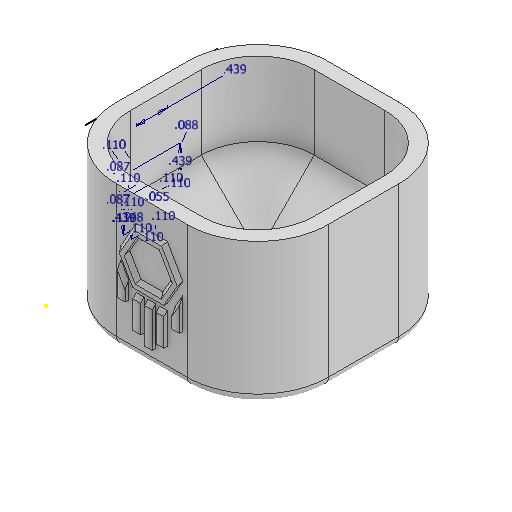
# Autodesk Inventor part: Hand Base
Saved by Autodesk Inventor 2025.1 (Build 291241020, 241B)
## iProperties
Created: 2025-01-03
Part Number: Hand Base
Material: Generic
Document SubType Name: Modeling
Designer: alexa
Density: 1 g/cm^3
Appearance: Default
Author: alexa
Autodesk Inventor part; units mm, degrees
ref_plane "YZ Plane" through (0, 0, 0) normal (1, 0, 0) x (0, 1, 0)
ref_plane "XZ Plane" through (0, 0, 0) normal (0, 1, 0) x (-1, 0, 0)
ref_plane "XY Plane" through (0, 0, 0) normal (0, 0, 1) x (1, 0, 0)
sketch "Sketch1" plane through (0, 0, 0) normal (0, 1, 0) x (-1, 0, 0)
  line L0 (0, 0) -> (-76.2, 0)
  line L1 (-76.2, 0) -> (-76.2, -76.2)
  line L2 (-76.2, -76.2) -> (0, -76.2)
  line L3 (0, -76.2) -> (0, 0)
  dimension "d0" = 76.2
  dimension "d1" = 76.2
  constraints: 8 end point, 2 parallel, 1 horizontal, 1 perpendicular
  measures "d0" distance of L2.end L0.start
  measures "d1" distance of L1.end L2.end
extrude "Extrusion1" add sketch "Sketch1" along normal blind 50.8
sketch "Sketch3" plane through (0, 0, 0) normal (0, -1, 0) x (1, 0, 0)
  line L0 (44.196, -54.102) -> (32.004, -54.102)
  line L1 (32.004, -54.102) -> (32.004, -22.098)
  line L2 (32.004, -22.098) -> (44.196, -22.098)
  line L3 (44.196, -22.098) -> (44.196, -54.102)
  line L4 (76.2, 0) -> (76.2, -76.2) projected
  line L5 (0, 0) -> (76.2, 0) projected
  line L6 (32.004, -40.132) -> (6.604, -40.132)
  line L7 (6.604, -40.132) -> (6.604, -36.068)
  line L8 (6.604, -36.068) -> (32.004, -36.068)
  line L9 (32.004, -36.068) -> (32.004, -40.132)
  point P0 (44.196, -38.1)
  point P1 (76.2, -38.1)
  point P2 (38.1, -22.098)
  point P3 (38.1, 0)
  point P4 (6.604, -38.1)
  point P5 (32.004, -38.1)
  dimension "d10" = 32.004
  dimension "d11" = 12.192
  dimension "d12" = 25.4
  dimension "d13" = 4.064
  constraints: 16 end point, 6 midpoint, 4 parallel, 2 horizontal, 2 horizontal alignment, 2 perpendicular, 1 point on line, 1 vertical alignment
  measures "d10" distance of L2.end L0.start
  measures "d11" distance of L0.start L0.end
  measures "d12" distance of L6.start L6.end
  measures "d13" distance of L6.end L7.end
extrude "Extrusion3" add sketch "Sketch3" along normal blind 6.35
sketch "Sketch4" plane through (0, -6.35, 0) normal (0, -1, 0) x (1, 0, 0)
  line L0 (43.942, -49.022) -> (32.258, -49.022)
  line L1 (32.258, -49.022) -> (32.258, -27.178)
  line L2 (32.258, -27.178) -> (43.942, -27.178)
  line L3 (43.942, -27.178) -> (43.942, -49.022)
  line L4 (44.196, -54.102) -> (44.196, -22.098) projected
  line L5 (32.004, -54.102) -> (44.196, -54.102) projected
  point P0 (0, 0)
  point P1 (32.258, -38.1)
  point P2 (44.196, -38.1)
  point P3 (38.1, -49.022)
  point P4 (38.1, -54.102)
  dimension "d16" = 21.844
  dimension "d17" = 11.684
  constraints: 8 end point, 4 midpoint, 2 parallel, 1 horizontal, 1 horizontal alignment, 1 perpendicular, 1 vertical alignment
  measures "d16" distance of L0.end L1.end
  measures "d17" distance between parallel lines of L1 L3
extrude "Extrusion4" add sketch "Sketch4" along normal blind 12.7
fillet "Fillet1" radius 25.4 4 edges at (0, 25.4, -76.2) (0, 25.4, 0) (76.2, 25.4, -76.2) (76.2, 25.4, 0)
sketch "Sketch5" plane through (0, 50.8, 0) normal (0, 1, 0) x (1, 0, 0)
  arc A0 (50.8, 0) -> (76.2, 25.4) centre (50.8, 25.4) ccw projected
  line L0 (76.2, 25.4) -> (76.2, 50.8) projected
  arc A1 (76.2, 50.8) -> (50.8, 76.2) centre (50.8, 50.8) ccw projected
  line L1 (50.8, 76.2) -> (25.4, 76.2) projected
  arc A2 (25.4, 76.2) -> (0, 50.8) centre (25.4, 50.8) ccw projected
  line L2 (0, 50.8) -> (0, 25.4) projected
  arc A3 (0, 25.4) -> (25.4, 0) centre (25.4, 25.4) ccw projected
  line L3 (25.4, 0) -> (50.8, 0) projected
  arc A4 (25.4, 71.12) -> (5.08, 50.8) centre (25.4, 50.8) ccw
  line L4 (25.4, 71.12) -> (50.8, 71.12)
  arc A5 (71.12, 50.8) -> (50.8, 71.12) centre (50.8, 50.8) ccw
  line L5 (71.12, 50.8) -> (71.12, 25.4)
  arc A6 (50.8, 5.08) -> (71.12, 25.4) centre (50.8, 25.4) ccw
  line L6 (50.8, 5.08) -> (25.4, 5.08)
  arc A7 (5.08, 25.4) -> (25.4, 5.08) centre (25.4, 25.4) ccw
  line L7 (5.08, 25.4) -> (5.08, 50.8)
  point P0 (0, 0)
  point P1 (38.1, 76.2)
  dimension "d21" = 5.08
  constraints: 8 end point, 8 point on circle, 4 centre point, 1 midpoint, 7 other
  measures "d21" distance from line of point (38.1, 76.2) L4
extrude "Extrusion5" cut sketch "Sketch5" against normal blind 45.72 contours L4 A5 L5 A6 L6 A7 L7 A4
fillet "Fillet2" radius 3.175 8 edges at (0, 0, -38.1) (7.4395, 0, -7.4395) (38.1, 0, 0) (68.7605, 0, -7.4395) (76.2, 0, -38.1) (68.7605, 0, -68.7605) (38.1, 0, -76.2) (7.4395, 0, -68.7605)
chamfer "Chamfer1" distance 19.05 angle 45 8 edges at (38.1, 5.08, -5.08) (11.0316, 5.08, -11.0316) (5.08, 5.08, -38.1) (11.0316, 5.08, -65.1684) (38.1, 5.08, -71.12) (65.1684, 5.08, -65.1684) (71.12, 5.08, -38.1) (65.1684, 5.08, -11.0316)
sketch "Sketch6" plane through (0, 50.8, -50.8) normal (-1, 0, 0) x (0, 0, 1)
  line L0 (7.2288, -10.0054) -> (18.3794, -10.0054)
  line L1 (18.3794, -10.0054) -> (23.9547, -19.6621)
  line L2 (23.9547, -19.6621) -> (18.3794, -29.3188)
  line L3 (18.3794, -29.3188) -> (7.2288, -29.3188)
  line L4 (7.2288, -29.3188) -> (1.6535, -19.6621)
  line L5 (1.6535, -19.6621) -> (7.2288, -10.0054)
  line L6 (16.7677, -26.5271) -> (20.7312, -19.6621)
  line L7 (20.7312, -19.6621) -> (16.7677, -12.797)
  line L8 (16.7677, -12.797) -> (8.8406, -12.797)
  line L9 (8.8406, -12.797) -> (4.877, -19.6621)
  line L10 (4.877, -19.6621) -> (8.8406, -26.5271)
  line L11 (8.8406, -26.5271) -> (16.7677, -26.5271)
  line L12 (23.9558, -24.0955) -> (23.9558, -35.2397)
  line L13 (23.9558, -35.2397) -> (21.1698, -35.2397)
  line L14 (21.1698, -35.2397) -> (21.1698, -28.9211)
  line L15 (21.1698, -28.9211) -> (23.9558, -24.0955)
  line L16 (18.3837, -42.6806) -> (15.5977, -42.6806)
  line L17 (15.5977, -42.6806) -> (15.5977, -31.5364)
  line L18 (7.2396, -31.5364) -> (7.2396, -42.6806)
  line L19 (7.2396, -42.6806) -> (10.0256, -42.6806)
  line L20 (10.0256, -42.6806) -> (10.0256, -31.5364)
  line L21 (1.6675, -24.1328) -> (1.6675, -35.2397)
  line L22 (1.6675, -35.2397) -> (4.4535, -35.2397)
  line L23 (4.4535, -35.2397) -> (4.4535, -28.9583)
  line L24 (4.4535, -28.9583) -> (1.6675, -24.1328)
  line L25 (14.2047, -45.4666) -> (14.2047, -31.5364)
  line L26 (14.2047, -31.5364) -> (11.4186, -31.5364)
  line L27 (11.4186, -31.5364) -> (11.4186, -45.4666)
  line L28 (11.4186, -45.4666) -> (14.2047, -45.4666)
  line L29 (10.0256, -31.5364) -> (7.2396, -31.5364)
  line L30 (15.5977, -42.6806) -> (14.2047, -42.6806) construction
  line L31 (10.0256, -42.6806) -> (11.4186, -42.6806) construction
  line L32 (18.3837, -42.6806) -> (18.3837, -31.5364)
  line L33 (18.3837, -31.5364) -> (15.5977, -31.5364)
  line L34 (12.8041, -44.5678) -> (12.8041, -1.5402) construction
  line L35 (36.5346, -1.5402) -> (-10.9264, -1.5402)
  point P0 (50.8, -50.8)
  point P1 (12.8041, -19.6621)
  dimension "d28" = 11.1506
  dimension "d29" = 2.7916
  dimension "d30" = 2.2177
  dimension "d31" = 2.2232
  dimension "d32" = 2.786
  dimension "d33" = 2.786
  dimension "d34" = 2.786
  dimension "d35" = 2.786
  dimension "d36" = 2.2177
  dimension "d37" = 11.1441
  dimension "d38" = 11.1441
  dimension "d39" = 13.9302
  dimension "d40" = 2.786
  dimension "d41" = 2.786
  dimension "d42" = 2.786
  dimension "d43" = 1.393
  dimension "d44" = 2.7903
  constraints: 72 end point, 8 perpendicular, 8 point on line, 5 parallel, 3 collinear, 1 midpoint, 1 vertical, 18 other
  measures "d28" distance of L5.end L0.end
  measures "d29" distance between parallel lines of L2 L6
  measures "d30" distance between parallel lines of L15 L2
  measures "d31" distance between parallel lines of L24 L4
  measures "d32" distance between parallel lines of L14 L12
  measures "d33" distance between parallel lines of L21 L23
  measures "d34" distance between parallel lines of L18 L20
  measures "d35" distance between parallel lines of L25 L27
  measures "d36" distance between parallel lines of L33 L3
  measures "d37" distance between parallel lines of L16 L33
  measures "d38" distance from line of L13 L15.end
  measures "d39" distance between parallel lines of L28 L26
  measures "d40" distance between parallel lines of L32 L17
  measures "d41" distance between parallel lines of L32 L14
  measures "d42" distance between parallel lines of L23 L18
  measures "d43" distance between parallel lines of L27 L20
  measures "d44" horizontal distance of L2.end L14.end
sketch "Sketch7" plane through (25.4, 50.8, 0) normal (0, 0, 1) x (1, 0, 0)
  line L0 (4.3171, -27.8388) -> (1.5311, -23.0133)
  line L1 (1.5311, -23.0133) -> (1.5311, -34.1202)
  line L2 (4.7406, -18.5426) -> (8.7041, -25.4077)
  line L3 (7.0924, -28.1993) -> (1.5171, -18.5426)
  line L4 (12.6677, -47.791) -> (12.6677, -4.9445) construction
  line L5 (8.7041, -11.6775) -> (4.7406, -18.5426)
  line L6 (1.5171, -18.5426) -> (7.0924, -8.8859)
  line L7 (1.5311, -34.1202) -> (4.3171, -34.1202)
  line L8 (4.3171, -34.1202) -> (4.3171, -27.8388)
  line L9 (16.6312, -25.4077) -> (20.5948, -18.5426)
  line L10 (23.8183, -18.5426) -> (18.243, -28.1993)
  line L11 (18.243, -28.1993) -> (7.0924, -28.1993)
  line L12 (7.0924, -8.8859) -> (18.243, -8.8859)
  line L13 (18.243, -8.8859) -> (23.8183, -18.5426)
  line L14 (84.753, -4.9445) -> (-59.4176, -4.9445)
  line L15 (16.6312, -11.6775) -> (8.7041, -11.6775)
  line L16 (8.7041, -25.4077) -> (16.6312, -25.4077)
  line L17 (20.5948, -18.5426) -> (16.6312, -11.6775)
  line L18 (21.0333, -34.1202) -> (21.0333, -27.8016)
  line L19 (21.0333, -27.8016) -> (23.8194, -22.976)
  line L20 (23.8194, -34.1202) -> (21.0333, -34.1202)
  line L21 (23.8194, -22.976) -> (23.8194, -34.1202)
  line L22 (18.2473, -41.5611) -> (15.4613, -41.5611)
  line L23 (15.4613, -41.5611) -> (15.4613, -30.4169)
  line L24 (14.0682, -30.4169) -> (11.2822, -30.4169)
  line L25 (18.2473, -30.4169) -> (15.4613, -30.4169)
  line L26 (9.8892, -30.4169) -> (7.1032, -30.4169)
  line L27 (7.1032, -30.4169) -> (7.1032, -41.5611)
  line L28 (7.1032, -41.5611) -> (9.8892, -41.5611)
  line L29 (18.2473, -41.5611) -> (18.2473, -30.4169)
  line L30 (15.4613, -41.5611) -> (14.0682, -41.5611) construction
  line L31 (9.8892, -41.5611) -> (9.8892, -30.4169)
  line L32 (9.8892, -41.5611) -> (11.2822, -41.5611) construction
  line L33 (14.0682, -44.3471) -> (14.0682, -30.4169)
  line L34 (11.2822, -30.4169) -> (11.2822, -44.3471)
  line L35 (11.2822, -44.3471) -> (14.0682, -44.3471)
  point P0 (-25.4, -50.8)
  point P1 (2.3088, -54.2043)
  point P2 (12.6677, -18.5426)
  dimension "d45" = 11.1506
  dimension "d46" = 2.7916
  dimension "d47" = 2.2177
  dimension "d48" = 2.2232
  dimension "d49" = 2.786
  dimension "d50" = 2.786
  dimension "d51" = 2.786
  dimension "d52" = 2.786
  dimension "d53" = 2.2177
  dimension "d54" = 11.1441
  dimension "d55" = 11.1441
  dimension "d56" = 13.9302
  dimension "d57" = 2.786
  dimension "d58" = 2.786
  dimension "d59" = 2.786
  dimension "d60" = 1.393
  dimension "d61" = 2.7903
  constraints: 72 end point, 8 perpendicular, 8 point on line, 5 parallel, 3 collinear, 1 midpoint, 1 vertical, 18 other
  measures "d45" distance of L6.end L13.start
  measures "d46" distance between parallel lines of L10 L9
  measures "d47" distance between parallel lines of L19 L10
  measures "d48" distance between parallel lines of L0 L3
  measures "d49" distance between parallel lines of L18 L21
  measures "d50" distance between parallel lines of L1 L8
  measures "d51" distance between parallel lines of L27 L31
  measures "d52" distance between parallel lines of L33 L34
  measures "d53" distance between parallel lines of L25 L11
  measures "d54" distance between parallel lines of L22 L25
  measures "d55" distance from line of L20 L19.end
  measures "d56" distance between parallel lines of L35 L24
  measures "d57" distance between parallel lines of L29 L23
  measures "d58" distance between parallel lines of L29 L18
  measures "d59" distance between parallel lines of L8 L27
  measures "d60" distance between parallel lines of L34 L31
  measures "d61" horizontal distance of L10.end L19.start
extrude "Extrusion6" add sketch "Sketch7" along normal blind 1.27
chamfer "Chamfer2" distance 1.27 angle 45 11 edges at (47.8264, 25.4112, 1.27) (42.2543, 20.3831, 1.27) (38.0752, 20.3831, 1.27) (33.8962, 20.3831, 1.27) (28.3241, 25.3739, 1.27) (32.1224, 28.8249, 1.27) (38.0677, 25.3923, 1.27) (44.013, 28.8249, 1.27) (46.4306, 37.0858, 1.27) (38.0677, 41.9141, 1.27) (29.7047, 37.0858, 1.27)
body "Solid1"
